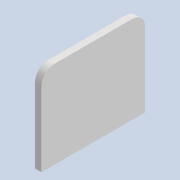
# Autodesk Inventor part: fingertip lid 5
Saved by Autodesk Inventor 2020 (Build 240168000, 168)
## iProperties
Created: 2020-01-28
Part Number: fingertip lid 5
Material: Generic
Document SubType Name: Modeling
Designer: kaipa
Density: 1 g/cm^3
Appearance: Default
Author: kaipa
Autodesk Inventor part; units mm, degrees
ref_plane "YZ Plane" through (0, 0, 0) normal (1, 0, 0) x (0, 1, 0)
ref_plane "XZ Plane" through (0, 0, 0) normal (0, 1, 0) x (-1, 0, 0)
ref_plane "XY Plane" through (0, 0, 0) normal (0, 0, 1) x (1, 0, 0)
sketch "Sketch1" plane through (0, 0, 0) normal (1, 0, 0) x (0, 1, 0)
  line L0 (6.75, 8) -> (-6.75, 8)
  line L1 (-6.75, 8) -> (-6.75, -8)
  line L2 (-6.75, -8) -> (6.75, -8)
  line L3 (6.75, -8) -> (6.75, 8)
  point P0 (0, 0)
  dimension "d0" = 16
  dimension "d1" = 13.5
  dimension "d2" = 6.75
  dimension "d3" = 8
  constraints: 8 end point, 2 parallel, 1 horizontal, 1 perpendicular
  measures "d0" distance of L0.end L1.end
  measures "d1" distance of L0.start L0.end
  measures "d2" distance from line of point (0, 0) L1
  measures "d3" distance from line of L2 point (0, 0)
extrude "Extrusion1" add sketch "Sketch1" along normal blind 1
fillet "Fillet1" radius 2 2 edges at (0.5, 6.75, 8) (0.5, 6.75, -8)
equation "\"d2\" = 0.5 * d1"
equation "\"d3\" = 0.5 * d0"
body "Solid1"
